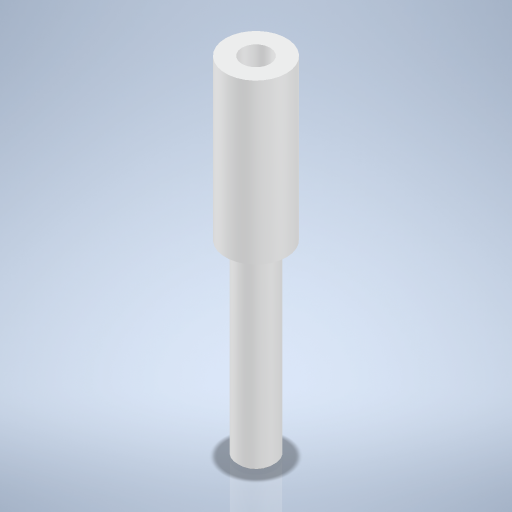
# Autodesk Inventor part: 202 Welle
Saved by Autodesk Inventor 2024 (Build 280153000, 153)
## iProperties
Created: 2024-07-12
Part Number: 202 Welle
Material: Aluminium 6061
Document SubType Name: Modeling
Designer: ffogue
Density: 2.7 g/cm^3
Appearance: Aluminium - flach
Author: ffogue
Autodesk Inventor part; units mm, degrees
ref_plane "YZ Plane" through (0, 0, 0) normal (1, 0, 0) x (0, 1, 0)
ref_plane "XZ Plane" through (0, 0, 0) normal (0, 1, 0) x (-1, 0, 0)
ref_plane "XY Plane" through (0, 0, 0) normal (0, 0, 1) x (1, 0, 0)
sketch "Skizze2" plane through (0, 0, 0) normal (0, 1, 0) x (-1, 0, 0)
  line L0 (0, 0) -> (6.5, 0)
  line L1 (6.5, 0) -> (6.5, -34)
  line L2 (6.5, -34) -> (4, -34)
  line L3 (4, -34) -> (4, -74)
  line L4 (4, -74) -> (0, -74)
  line L5 (0, -74) -> (0, 0)
  dimension "d3" = 13
  dimension "d4" = 8
  dimension "d5" = 34
  dimension "d6" = 40
  constraints: 12 end point, 5 perpendicular, 1 horizontal
  measures "d3" diameter of L1 L5
  measures "d4" diameter of L3 L5
  measures "d5" distance between parallel lines of L2 L0
  measures "d6" distance between parallel lines of L4 L2
revolve "Umdrehung1" add sketch "Skizze2" angle 360 about axis through (0, 0, -74) along (0, 0, 1)
chamfer "Fasen1" distance 0.6 angle 45 1 edges at (4, 0, -74)
sketch "Skizze3" plane through (0, 0, 0) normal (0, 0, 1) x (1, 0, 0)
  circle A0 centre (0, 0) radius 6.5 projected
  point P0 (0, 0)
  constraints: 1 coincident
hole "Bohrung1" at (0, 0, 0) direction (0, 0, -1) diameter 6 depth 34
